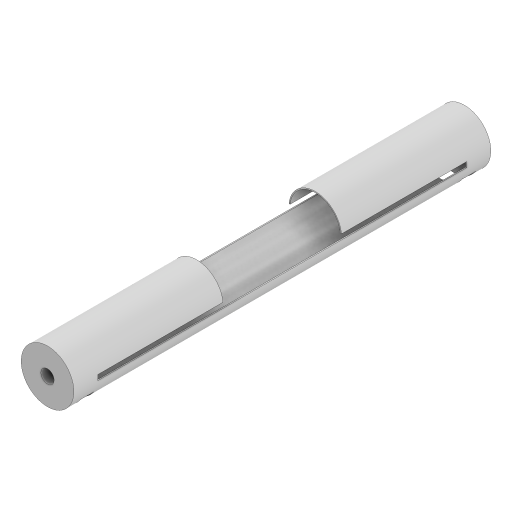
# Autodesk Inventor part: GUIA_DE_OBJETO
Saved by Autodesk Inventor 2024 (Build 280153000, 153)
## iProperties
Created: 2024-05-26
Part Number: GUIA_DE_OBJETO
Material: Generic
Document SubType Name: Modeling
Designer: Jhuliams
Density: 1 g/cm^3
Appearance: Default
Author: Jhuliams
Autodesk Inventor part; units mm, degrees
ref_plane "YZ Plane" through (0, 0, 0) normal (1, 0, 0) x (0, 1, 0)
ref_plane "XZ Plane" through (0, 0, 0) normal (0, 1, 0) x (-1, 0, 0)
ref_plane "XY Plane" through (0, 0, 0) normal (0, 0, 1) x (1, 0, 0)
sketch "Sketch1" plane through (0, 0, 0) normal (0, 0, 1) x (1, 0, 0)
  circle A0 centre (0, 0) radius 60
  line L0 (-60, 0) -> (60, 0)
  circle A1 centre (0, 0) radius 57.5
  point P0 (57.5, 0)
  point P1 (-57.5, 0)
  dimension "d0" = 120
  dimension "d2" = 115
  constraints: 2 centre point, 2 coincident, 2 end point, 2 point on circle, 1 horizontal
  measures "d0" diameter of A0
  measures "d2" diameter of A1
extrude "Extrusion1" add sketch "Sketch1" along normal mid plane 900 contours L0 A1 A0 | A0 L0 A1
sketch "Sketch3" plane through (0, 0, 450) normal (0, 0, 1) x (1, 0, 0)
  circle A0 centre (0, 0) radius 60
  dimension "d5" = 120
  constraints: 1 centre point, 1 coincident
  measures "d5" diameter of A0
extrude "Extrusion2" add sketch "Sketch3" along normal blind 5
sketch "Sketch4" plane through (0, 0, -450) normal (0, 0, -1) x (-1, 0, 0)
  circle A0 centre (0, 0) radius 60
  dimension "d8" = 120
  constraints: 1 centre point, 1 coincident
  measures "d8" diameter of A0
extrude "Extrusion3" add sketch "Sketch4" along normal blind 5
sketch "Sketch5" plane through (0, 0, 0) normal (0, 1, 0) x (-1, 0, 0)
  line L0 (0, 0) -> (0, 435) construction
  line L1 (50, 450) -> (-50, 450)
  line L2 (-50, 450) -> (-50, 420)
  line L3 (-50, 420) -> (50, 420)
  line L4 (50, 420) -> (50, 450)
  line L5 (50, 450) -> (-50, 420) construction
  line L6 (-50, 450) -> (50, 420) construction
  line L7 (0, 0) -> (20, 0) construction
  line L8 (50, -450) -> (-50, -450)
  line L9 (-50, -450) -> (-50, -420)
  line L10 (-50, -420) -> (50, -420)
  line L11 (50, -420) -> (50, -450)
  line L12 (50, -450) -> (-50, -420) construction
  line L13 (-50, -450) -> (50, -420) construction
  point P0 (0, -435)
  dimension "d11" = 435
  dimension "d12" = 100
  dimension "d13" = 30
  dimension "d14" = 20
  constraints: 28 end point, 5 symmetric about line, 2 horizontal, 2 midpoint, 2 parallel, 1 perpendicular, 1 vertical
  measures "d11" distance of L0.start L0.end
  measures "d12" distance of L3.end L2.end
  measures "d13" distance of L2.end L1.end
  measures "d14" distance of L0.start L7.end
extrude "Extrusion4" cut sketch "Sketch5" against normal blind 80
sketch "Sketch6" plane through (0, 0, 0) normal (0, 1, 0) x (-1, 0, 0)
  line L0 (60, 135) -> (-60, 135)
  line L1 (-60, 135) -> (-60, -135)
  line L2 (-60, -135) -> (60, -135)
  line L3 (60, -135) -> (60, 135)
  line L4 (60, 135) -> (-60, -135) construction
  line L5 (-60, 135) -> (60, -135) construction
  point P0 (0, 0)
  dimension "d17" = 120
  dimension "d18" = 270
  constraints: 12 end point, 2 midpoint, 2 parallel, 1 horizontal, 1 perpendicular
  measures "d17" distance of L2.end L1.end
  measures "d18" distance of L1.end L0.end
extrude "Extrusion5" cut sketch "Sketch6" along normal blind 100
sketch "Sketch7" plane through (0, 0, 0) normal (1, 0, 0) x (0, 1, 0)
  line L0 (6, 420) -> (-6, 420)
  line L1 (-6, 420) -> (-6, -420)
  line L2 (-6, -420) -> (6, -420)
  line L3 (6, -420) -> (6, 420)
  line L4 (6, 420) -> (-6, -420) construction
  line L5 (-6, 420) -> (6, -420) construction
  point P0 (0, 0)
  dimension "d21" = 12
  dimension "d22" = 840
  constraints: 12 end point, 2 midpoint, 2 parallel, 1 horizontal, 1 perpendicular
  measures "d21" distance of L2.end L1.end
  measures "d22" distance of L1.end L0.end
extrude "Extrusion6" cut sketch "Sketch7" along normal mid plane 200
sketch "Sketch8" plane through (0, 0, 455) normal (0, 0, 1) x (1, 0, 0)
  circle A0 centre (0, 0) radius 15
  dimension "d25" = 30
  constraints: 1 centre point, 1 coincident
  measures "d25" diameter of A0
extrude "Extrusion7" cut sketch "Sketch8" against normal blind 1000
sketch "Sketch9" plane through (0, 0, 455) normal (0, 0, 1) x (1, 0, 0)
  circle A0 centre (0, 0) radius 15 projected
  circle A1 centre (0, 0) radius 60 projected
extrude "Extrusion8" add sketch "Sketch9" along normal blind 20
sketch "Sketch10" plane through (0, 0, -455) normal (0, 0, -1) x (-1, 0, 0)
  circle A0 centre (0, 0) radius 15 projected
  circle A1 centre (0, 0) radius 60 projected
extrude "Extrusion9" add sketch "Sketch10" along normal blind 20
body "Solid1"
